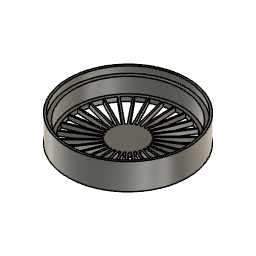
Fan front body (Autodesk Fusion 360 design; units mm, degrees)
Autodesk Fusion 360 part; units mm, degrees
sketch "Sketch1" plane through (0, 0, 0) normal (0, 0, 1) x (1, 0, 0) in component "P1"
  circle A0 centre (0, 0) radius 25
  circle A1 centre (0, 0) radius 137.5
  line L0 (-92.5259, 72.6579) -> (-105.6105, 51.8329)
  line L1 (-105.6105, 51.8329) -> (-114.0793, 28.7426)
  line L2 (-114.0793, 28.7426) -> (-117.5623, 4.3961)
  line L3 (-117.5623, 4.3961) -> (-115.9073, -20.1426)
  line L4 (-115.9073, -20.1426) -> (-109.1866, -43.8009)
  line L5 (-109.1866, -43.8009) -> (-97.6939, -65.5449)
  line L6 (-97.6939, -65.5449) -> (-81.9315, -84.4243)
  line L7 (-81.9315, -84.4243) -> (-62.5883, -99.6139)
  line L8 (-62.5883, -99.6139) -> (-40.5097, -110.4499)
  line L9 (-40.5097, -110.4499) -> (-16.6606, -116.4588)
  line L10 (-16.6606, -116.4588) -> (7.9166, -117.3778)
  line L11 (7.9166, -117.3778) -> (32.1478, -113.1669)
  line L12 (32.1478, -113.1669) -> (54.974, -104.01)
  line L13 (54.974, -104.01) -> (75.3976, -90.3074)
  line L14 (75.3976, -90.3074) -> (92.5259, -72.6579)
  line L15 (92.5259, -72.6579) -> (105.6105, -51.8329)
  line L16 (105.6105, -51.8329) -> (114.0793, -28.7426)
  line L17 (114.0793, -28.7426) -> (117.5623, -4.3961)
  line L18 (117.5623, -4.3961) -> (115.9073, 20.1426)
  line L19 (115.9073, 20.1426) -> (109.1866, 43.8009)
  line L20 (109.1866, 43.8009) -> (97.6939, 65.5449)
  line L21 (97.6939, 65.5449) -> (81.9315, 84.4243)
  line L22 (81.9315, 84.4243) -> (62.5883, 99.6139)
  line L23 (62.5883, 99.6139) -> (40.5097, 110.4499)
  line L24 (40.5097, 110.4499) -> (16.6606, 116.4588)
  line L25 (16.6606, 116.4588) -> (-7.9166, 117.3778)
  line L26 (-7.9166, 117.3778) -> (-32.1478, 113.1669)
  line L27 (-32.1478, 113.1669) -> (-54.974, 104.01)
  line L28 (-54.974, 104.01) -> (-75.3976, 90.3074)
  line L29 (-75.3976, 90.3074) -> (-92.5259, 72.6579)
  line L30 (-114.0793, 28.7426) -> (-117.5623, 4.3961)
  line L31 (-117.5623, 4.3961) -> (-115.9073, -20.1426)
  line L32 (-115.9073, -20.1426) -> (-109.1866, -43.8009)
  line L33 (-109.1866, -43.8009) -> (-97.6939, -65.5449)
  line L34 (-97.6939, -65.5449) -> (-81.9315, -84.4243)
  line L35 (-81.9315, -84.4243) -> (-62.5883, -99.6139)
  line L36 (-62.5883, -99.6139) -> (-40.5097, -110.4499)
  line L37 (-40.5097, -110.4499) -> (-16.6606, -116.4588)
  line L38 (-16.6606, -116.4588) -> (7.9166, -117.3778)
  line L39 (7.9166, -117.3778) -> (32.1478, -113.1669)
  line L40 (32.1478, -113.1669) -> (54.974, -104.01)
  line L41 (54.974, -104.01) -> (75.3976, -90.3074)
  line L42 (75.3976, -90.3074) -> (92.5259, -72.6579)
  line L43 (92.5259, -72.6579) -> (105.6105, -51.8329)
  line L44 (105.6105, -51.8329) -> (114.0793, -28.7426)
  line L45 (114.0793, -28.7426) -> (117.5623, -4.3961)
  line L46 (117.5623, -4.3961) -> (115.9073, 20.1426)
  line L47 (115.9073, 20.1426) -> (109.1866, 43.8009)
  line L48 (109.1866, 43.8009) -> (97.6939, 65.5449)
  line L49 (97.6939, 65.5449) -> (81.9315, 84.4243)
  line L50 (81.9315, 84.4243) -> (62.5883, 99.6139)
  line L51 (62.5883, 99.6139) -> (40.5097, 110.4499)
  line L52 (40.5097, 110.4499) -> (16.6606, 116.4588)
  line L53 (16.6606, 116.4588) -> (-7.9166, 117.3778)
  line L54 (-7.9166, 117.3778) -> (-32.1478, 113.1669)
  line L55 (-32.1478, 113.1669) -> (-54.974, 104.01)
  line L56 (-54.974, 104.01) -> (-75.3976, 90.3074)
  line L57 (-75.3976, 90.3074) -> (-92.5259, 72.6579)
  line L58 (-92.5259, 72.6579) -> (-105.6105, 51.8329)
  line L59 (-105.6105, 51.8329) -> (-114.0793, 28.7426)
  line L60 (-31.5682, 24.9223) -> (-36.06, 17.8143)
  line L61 (-36.06, 17.8143) -> (-38.9758, 9.9277)
  line L62 (-38.9758, 9.9277) -> (-40.1882, 1.6072)
  line L63 (-40.1882, 1.6072) -> (-39.6442, -6.7835)
  line L64 (-39.6442, -6.7835) -> (-37.3675, -14.8777)
  line L65 (-37.3675, -14.8777) -> (-33.4576, -22.3218)
  line L66 (-33.4576, -22.3218) -> (-28.0856, -28.7902)
  line L67 (-28.0856, -28.7902) -> (-21.486, -34.0004)
  line L68 (-21.486, -34.0004) -> (-13.9474, -37.7246)
  line L69 (-13.9474, -37.7246) -> (-5.7992, -39.8001)
  line L70 (-5.7992, -39.8001) -> (2.6024, -40.1361)
  line L71 (2.6024, -40.1361) -> (10.8903, -38.7179)
  line L72 (10.8903, -38.7179) -> (18.7022, -35.6076)
  line L73 (18.7022, -35.6076) -> (25.6968, -30.9411)
  line L74 (25.6968, -30.9411) -> (31.5682, -24.9223)
  line L75 (31.5682, -24.9223) -> (36.06, -17.8143)
  line L76 (36.06, -17.8143) -> (38.9758, -9.9277)
  line L77 (38.9758, -9.9277) -> (40.1882, -1.6072)
  line L78 (40.1882, -1.6072) -> (39.6442, 6.7835)
  line L79 (39.6442, 6.7835) -> (37.3675, 14.8777)
  line L80 (37.3675, 14.8777) -> (33.4576, 22.3218)
  line L81 (33.4576, 22.3218) -> (28.0856, 28.7902)
  line L82 (28.0856, 28.7902) -> (21.486, 34.0004)
  line L83 (21.486, 34.0004) -> (13.9474, 37.7246)
  line L84 (13.9474, 37.7246) -> (5.7992, 39.8001)
  line L85 (5.7992, 39.8001) -> (-2.6024, 40.1361)
  line L86 (-2.6024, 40.1361) -> (-10.8903, 38.7179)
  line L87 (-10.8903, 38.7179) -> (-18.7022, 35.6076)
  line L88 (-18.7022, 35.6076) -> (-25.6968, 30.9411)
  line L89 (-25.6968, 30.9411) -> (-31.5682, 24.9223)
  line L90 (-105.6105, 51.8329) -> (-36.06, 17.8143)
  line L91 (-114.0793, 28.7426) -> (-38.9758, 9.9277)
  line L92 (-117.5623, 4.3961) -> (-40.1882, 1.6072)
  line L93 (-115.9073, -20.1426) -> (-39.6442, -6.7835)
  line L94 (-109.1866, -43.8009) -> (-37.3675, -14.8777)
  line L95 (-97.6939, -65.5449) -> (-33.4576, -22.3218)
  line L96 (-28.0856, -28.7902) -> (-81.9315, -84.4243)
  line L97 (-62.5883, -99.6139) -> (-21.486, -34.0004)
  line L98 (-13.9474, -37.7246) -> (-40.5097, -110.4499)
  line L99 (-5.7992, -39.8001) -> (-16.6606, -116.4588)
  line L100 (2.6024, -40.1361) -> (7.9166, -117.3778)
  line L101 (10.8903, -38.7179) -> (32.1478, -113.1669)
  line L102 (18.7022, -35.6076) -> (54.974, -104.01)
  line L103 (25.6968, -30.9411) -> (75.3976, -90.3074)
  line L104 (31.5682, -24.9223) -> (92.5259, -72.6579)
  line L105 (36.06, -17.8143) -> (105.6105, -51.8329)
  line L106 (38.9758, -9.9277) -> (114.0793, -28.7426)
  line L107 (40.1882, -1.6072) -> (117.5623, -4.3961)
  line L108 (39.6442, 6.7835) -> (115.9073, 20.1426)
  line L109 (37.3675, 14.8777) -> (109.1866, 43.8009)
  line L110 (33.4576, 22.3218) -> (97.6939, 65.5449)
  line L111 (28.0856, 28.7902) -> (81.9315, 84.4243)
  line L112 (21.486, 34.0004) -> (62.5883, 99.6139)
  line L113 (13.9474, 37.7246) -> (40.5097, 110.4499)
  line L114 (16.6606, 116.4588) -> (5.7992, 39.8001)
  line L115 (-7.9166, 117.3778) -> (-2.6024, 40.1361)
  line L116 (-32.1478, 113.1669) -> (-10.8903, 38.7179)
  line L117 (-54.974, 104.01) -> (-18.7022, 35.6076)
  line L118 (-92.5259, 72.6579) -> (-31.5682, 24.9223)
  line L119 (-75.3976, 90.3074) -> (-25.6968, 30.9411)
  dimension "d1" = 50
  dimension "d6" = 275
  dimension "d7" = 117
  dimension "d8" = 40
  constraint coincident A0.centre A1.centre
  measures "d1" diameter of A0
  measures "d6" diameter of A1
  measures "d7" distance of A0.centre L29
  measures "d8" distance of A0.centre L89
sketch "Sketch2" plane through (0, 0, 0) normal (0, 0, 1) x (1, 0, 0) in component "P1"
  line L0 (-36.3108, 17.2975) -> (-39.1136, 9.3701)
  line L1 (-39.1136, 9.3701) -> (-40.2071, 1.0331)
  line L2 (-40.2071, 1.0331) -> (-39.5432, -7.349)
  line L3 (-39.5432, -7.349) -> (-37.1512, -15.4099)
  line L4 (-37.1512, -15.4099) -> (-33.1355, -22.7973)
  line L5 (-33.1355, -22.7973) -> (-27.6715, -29.1884)
  line L6 (-27.6715, -29.1884) -> (-20.9983, -34.3038)
  line L7 (-20.9983, -34.3038) -> (-13.4072, -37.9199)
  line L8 (-13.4072, -37.9199) -> (-5.2303, -39.8788)
  line L9 (-5.2303, -39.8788) -> (3.1753, -40.0948)
  line L10 (3.1753, -40.0948) -> (11.4421, -38.5584)
  line L11 (11.4421, -38.5584) -> (19.2088, -35.3369)
  line L12 (19.2088, -35.3369) -> (26.136, -30.571)
  line L13 (26.136, -30.571) -> (31.9209, -24.4689)
  line L14 (31.9209, -24.4689) -> (36.3108, -17.2975)
  line L15 (36.3108, -17.2975) -> (39.1136, -9.3701)
  line L16 (39.1136, -9.3701) -> (40.2071, -1.0331)
  line L17 (40.2071, -1.0331) -> (39.5432, 7.349)
  line L18 (39.5432, 7.349) -> (37.1512, 15.4099)
  line L19 (37.1512, 15.4099) -> (33.1355, 22.7973)
  line L20 (33.1355, 22.7973) -> (27.6715, 29.1884)
  line L21 (27.6715, 29.1884) -> (20.9983, 34.3038)
  line L22 (20.9983, 34.3038) -> (13.4072, 37.9199)
  line L23 (13.4072, 37.9199) -> (5.2303, 39.8788)
  line L24 (5.2303, 39.8788) -> (-3.1753, 40.0948)
  line L25 (-3.1753, 40.0948) -> (-11.4421, 38.5584)
  line L26 (-11.4421, 38.5584) -> (-19.2088, 35.3369)
  line L27 (-19.2088, 35.3369) -> (-26.136, 30.571)
  line L28 (-26.136, 30.571) -> (-31.9209, 24.4689)
  line L29 (-31.9209, 24.4689) -> (-36.3108, 17.2975)
  line L30 (-94.5441, 70.4382) -> (-34.1158, 20.8832)
  line L31 (-31.9209, 24.4689) -> (-91.7989, 73.5727)
  line L32 (-91.7989, 73.5727) -> (-94.5441, 70.4382)
  line L33 (-75.334, 90.2327) -> (-77.6493, 88.325)
  line L34 (-77.6493, 88.325) -> (-29.0285, 27.52)
  line L35 (-26.136, 30.571) -> (-75.334, 90.2327)
  line L36 (-94.5441, 70.4382) -> (-93.1715, 72.0054)
  line L37 (-57.7827, 102.4024) -> (-55.0494, 103.6389)
  line L38 (-55.0494, 103.6389) -> (-19.2088, 35.3369)
  line L39 (-22.6724, 32.9539) -> (-57.7827, 102.4024)
  line L40 (-32.148, 113.167) -> (-34.9624, 112.1282)
  line L41 (-34.9624, 112.1282) -> (-15.3254, 36.9477)
  line L42 (-11.4421, 38.5584) -> (-32.148, 113.167)
  line L43 (-3.1753, 40.0948) -> (-7.7901, 117.2299)
  line L44 (-7.7901, 117.2299) -> (-10.7847, 117.0508)
  line L45 (-10.7847, 117.0508) -> (-7.3087, 39.3266)
  line L46 (-3.1753, 40.0948) -> (-7.7901, 117.2299)
  line L47 (16.8251, 116.2807) -> (13.8251, 116.2807)
  line L48 (13.8251, 116.2807) -> (1.0275, 39.9868)
  line L49 (5.2303, 39.8788) -> (16.8251, 116.2807)
  line L50 (40.5383, 110.4147) -> (37.6703, 111.2947)
  line L51 (37.6703, 111.2947) -> (9.3188, 38.8994)
  line L52 (13.4072, 37.9199) -> (40.5383, 110.4147)
  line L53 (62.5134, 99.4538) -> (59.7037, 100.5053)
  line L54 (59.7037, 100.5053) -> (17.2027, 36.1118)
  line L55 (20.9983, 34.3038) -> (62.5134, 99.4538)
  line L56 (82, 84) -> (79.7982, 86.0377)
  line L57 (79.7982, 86.0377) -> (24.3349, 31.7461)
  line L58 (27.6715, 29.1884) -> (82, 84)
  line L59 (97.7404, 65.3757) -> (95.6097, 67.4876)
  line L60 (95.6097, 67.4876) -> (30.4035, 25.9928)
  line L61 (33.1355, 22.7973) -> (97.7404, 65.3757)
  line L62 (109.2924, 44.0865) -> (107.6415, 46.5914)
  line L63 (107.6415, 46.5914) -> (35.1433, 19.1036)
  line L64 (37.1512, 15.4099) -> (109.2924, 44.0865)
  line L65 (116, 20) -> (114.8918, 22.7878)
  line L66 (114.8918, 22.7878) -> (38.3472, 11.3794)
  line L67 (39.5432, 7.349) -> (116, 20)
  line L68 (117.789, -4.8117) -> (117.2992, -1.8519)
  line L69 (117.2992, -1.8519) -> (39.8752, 3.1579)
  line L70 (40.2071, -1.0331) -> (117.789, -4.8117)
  line L71 (114, -29) -> (114.4863, -26.0397)
  line L72 (114.4863, -26.0397) -> (39.6603, -5.2016)
  line L73 (39.1136, -9.3701) -> (114, -29)
  line L74 (105.7119, -51.9678) -> (106.4726, -49.0659)
  line L75 (106.4726, -49.0659) -> (37.7122, -13.3338)
  line L76 (36.3108, -17.2975) -> (105.7119, -51.9678)
  line L77 (92.7602, -72.7218) -> (94.1009, -70.038)
  line L78 (94.1009, -70.038) -> (34.1158, -20.8832)
  line L79 (31.9209, -24.4689) -> (92.7602, -72.7218)
  line L80 (75.4679, -90.2781) -> (77.7305, -88.3082)
  line L81 (77.7305, -88.3082) -> (29.0285, -27.52)
  line L82 (26.136, -30.571) -> (75.4679, -90.2781)
  line L83 (32.3249, -113.2073) -> (35.0941, -112.0535)
  line L84 (35.0941, -112.0535) -> (15.3254, -36.9477)
  line L85 (11.4421, -38.5584) -> (32.3249, -113.2073)
  line L86 (55, -104) -> (57.5118, -102.3596)
  line L87 (57.5118, -102.3596) -> (22.6724, -32.9539)
  line L88 (19.2088, -35.3369) -> (55, -104)
  line L89 (7.3087, -117.1355) -> (10.2582, -116.5873)
  line L90 (10.2582, -116.5873) -> (7.3087, -39.3266)
  line L91 (3.1753, -40.0948) -> (7.3087, -117.1355)
  line L92 (-16.4966, -116.6928) -> (-13.4966, -116.6928)
  line L93 (-13.4966, -116.6928) -> (-1.0275, -39.9868)
  line L94 (-5.2303, -39.8788) -> (-16.4966, -116.6928)
  line L95 (-40, -110) -> (-37.1974, -111.0702)
  line L96 (-37.1974, -111.0702) -> (-9.3188, -38.8994)
  line L97 (-13.4072, -37.9199) -> (-40, -110)
  line L98 (-62.5344, -99.65) -> (-59.7198, -100.6884)
  line L99 (-59.7198, -100.6884) -> (-17.2027, -36.1118)
  line L100 (-20.9983, -34.3038) -> (-62.5344, -99.65)
  line L101 (-82.0119, -84.3778) -> (-79.5062, -86.0276)
  line L102 (-79.5062, -86.0276) -> (-24.3349, -31.7461)
  line L103 (-27.6715, -29.1884) -> (-82.0119, -84.3778)
  line L104 (-97.7267, -65.5643) -> (-95.589, -67.6691)
  line L105 (-95.589, -67.6691) -> (-30.4035, -25.9928)
  line L106 (-33.1355, -22.7973) -> (-97.7267, -65.5643)
  line L107 (-109.2361, -44.1808) -> (-107.5799, -46.6822)
  line L108 (-107.5799, -46.6822) -> (-35.1433, -19.1036)
  line L109 (-37.1512, -15.4099) -> (-109.2361, -44.1808)
  line L110 (-116, -20) -> (-114.8879, -22.7863)
  line L111 (-114.8879, -22.7863) -> (-38.3472, -11.3794)
  line L112 (-39.5432, -7.349) -> (-116, -20)
  line L113 (-117.8376, 4.2071) -> (-117.3479, 1.2473)
  line L114 (-117.3479, 1.2473) -> (-39.8752, -3.1579)
  line L115 (-40.2071, 1.0331) -> (-117.8376, 4.2071)
  line L116 (-114.3122, 28.3563) -> (-114.4825, 25.3611)
  line L117 (-114.4825, 25.3611) -> (-39.6603, 5.2016)
  line L118 (-39.1136, 9.3701) -> (-114.3122, 28.3563)
  line L119 (-105.3224, 51.9766) -> (-106.1029, 49.0799)
  line L120 (-106.1029, 49.0799) -> (-37.7122, 13.3338)
  line L121 (-36.3108, 17.2975) -> (-105.3224, 51.9766)
  point P0 (-75.3976, 90.3074)
  point P1 (-92.5259, 72.6579)
  dimension "d9" = 40
  dimension "d10" = 3
  dimension "d11" = 3
  dimension "d12" = 3
  dimension "d13" = 3
  dimension "d14" = 3
  dimension "d16" = 3
  dimension "d17" = 3
  dimension "d18" = 3
  dimension "d19" = 3
  dimension "d20" = 3
  dimension "d21" = 3
  dimension "d22" = 3
  dimension "d23" = 3
  dimension "d24" = 3
  dimension "d25" = 3
  dimension "d26" = 3
  dimension "d27" = 3
  dimension "d28" = 3
  dimension "d29" = 3
  dimension "d30" = 3
  dimension "d31" = 3
  dimension "d32" = 3
  dimension "d33" = 3
  dimension "d34" = 3
  dimension "d35" = 3
  dimension "d36" = 3
  dimension "d37" = 3
  dimension "d38" = 3
  dimension "d39" = 3
  dimension "d40" = 3
  dimension "d41" = 3
  constraint midpoint L29 L30.end
  constraint parallel L30 L31
  constraint midpoint L28 L34.end
  constraint midpoint L32 L36.end
  constraint midpoint L27 L39.start
  constraint midpoint L26 L41.end
  constraint perpendicular L43 L44
  constraint midpoint L25 L45.end
  constraint horizontal L47
  constraint midpoint L24 L48.end
  constraint midpoint L23 L51.end
  constraint perpendicular L52 L53
  constraint midpoint L22 L54.end
  constraint midpoint L21 L57.end
  constraint perpendicular L58 L59
  constraint midpoint L20 L60.end
  constraint perpendicular L61 L62
  constraint midpoint L19 L63.end
  constraint perpendicular L64 L65
  constraint midpoint L18 L66.end
  constraint perpendicular L67 L68
  constraint midpoint L17 L69.end
  constraint midpoint L16 L72.end
  constraint perpendicular L73 L74
  constraint midpoint L15 L75.end
  constraint perpendicular L76 L77
  constraint midpoint L14 L78.end
  constraint midpoint L13 L81.end
  constraint midpoint L11 L84.end
  constraint midpoint L12 L87.end
  constraint parallel L10 L89
  constraint midpoint L10 L90.end
  constraint horizontal L92
  constraint midpoint L9 L93.end
  constraint midpoint L8 L96.end
  constraint perpendicular L97 L98
  constraint midpoint L7 L99.end
  constraint perpendicular L99 L101
  constraint midpoint L6 L102.end
  constraint perpendicular L103 L104
  constraint midpoint L5 L105.end
  constraint perpendicular L106 L107
  constraint midpoint L4 L108.end
  constraint perpendicular L109 L110
  constraint midpoint L3 L111.end
  constraint perpendicular L112 L113
  constraint midpoint L2 L114.end
  constraint perpendicular L114 L116
  constraint midpoint L1 L117.end
  constraint perpendicular L117 L119
  constraint midpoint L0 L120.end
  measures "d9" distance of origin L29
  measures "d10" distance of L33.start L33.end
  measures "d11" distance of L33.end P0
  measures "d12" distance of L30.start P1
  measures "d13" distance of L37.start L37.end
  measures "d14" distance of L40.start L40.end
  measures "d16" distance of L43.end L44.end
  measures "d17" distance of L47.start L47.end
  measures "d18" distance of L50.start L50.end
  measures "d19" distance of L53.start L53.end
  measures "d20" distance of L56.start L56.end
  measures "d21" distance of L59.start L59.end
  measures "d22" distance of L62.start L62.end
  measures "d23" distance of L65.start L65.end
  measures "d24" distance of L68.start L68.end
  measures "d25" distance of L71.start L71.end
  measures "d26" distance of L74.start L74.end
  measures "d27" distance of L77.start L77.end
  measures "d28" distance of L80.start L80.end
  measures "d29" distance of L83.start L83.end
  measures "d30" distance of L86.start L86.end
  measures "d31" distance of L89.start L89.end
  measures "d32" distance of L92.start L92.end
  measures "d33" distance of L95.start L95.end
  measures "d34" distance of L98.start L98.end
  measures "d35" distance of L101.start L101.end
  measures "d36" distance of L104.start L104.end
  measures "d37" distance of L107.start L107.end
  measures "d38" distance of L110.start L110.end
  measures "d39" distance of L113.start L113.end
  measures "d40" distance of L116.start L116.end
  measures "d41" distance of L119.start L119.end
extrude "Extrude1" add sketch "Sketch2" sketch "Sketch1" along normal blind 10 of sketch 2 contours A1 in component "P1"
sketch "Sketch3" plane through (0, 0, 10) normal (0, 0, 1) x (-1, 0, 0) in component "P1"
  line L0 (114.4294, -26.2951) -> (114.4825, -25.3611)
  line L1 (114.4825, -25.3611) -> (39.6603, -5.2016)
  line L2 (39.6603, -5.2016) -> (40.2071, -1.0331)
  line L3 (40.2071, -1.0331) -> (117.5488, -4.1953)
  line L4 (117.5488, -4.1953) -> (117.5623, -4.3961)
  line L5 (117.5623, -4.3961) -> (114.4294, -26.2951)
  line L6 (117.3513, -1.268) -> (117.3479, -1.2473)
  line L7 (117.3479, -1.2473) -> (39.8752, 3.1579)
  line L8 (39.8752, 3.1579) -> (39.5432, 7.349)
  line L9 (39.5432, 7.349) -> (115.9178, 19.9864)
  line L10 (115.9178, 19.9864) -> (117.3513, -1.268)
  line L11 (115.8188, 20.4539) -> (114.8879, 22.7863)
  line L12 (114.8879, 22.7863) -> (38.3472, 11.3794)
  line L13 (38.3472, 11.3794) -> (37.1512, 15.4099)
  line L14 (37.1512, 15.4099) -> (109.0294, 44.0983)
  line L15 (109.0294, 44.0983) -> (109.1866, 43.8009)
  line L16 (109.1866, 43.8009) -> (115.8188, 20.4539)
  line L17 (107.9951, 46.0551) -> (107.5799, 46.6822)
  line L18 (107.5799, 46.6822) -> (35.1433, 19.1036)
  line L19 (35.1433, 19.1036) -> (33.1355, 22.7973)
  line L20 (33.1355, 22.7973) -> (97.6947, 65.5432)
  line L21 (97.6947, 65.5432) -> (107.9951, 46.0551)
  line L22 (97.451, 65.8357) -> (95.589, 67.6691)
  line L23 (95.589, 67.6691) -> (30.4035, 25.9928)
  line L24 (30.4035, 25.9928) -> (27.6715, 29.1884)
  line L25 (27.6715, 29.1884) -> (81.9893, 84.355)
  line L26 (81.9893, 84.355) -> (97.451, 65.8357)
  line L27 (81.8802, 84.4645) -> (79.5062, 86.0276)
  line L28 (79.5062, 86.0276) -> (24.3349, 31.7461)
  line L29 (24.3349, 31.7461) -> (20.9983, 34.3038)
  line L30 (20.9983, 34.3038) -> (62.5297, 99.6426)
  line L31 (62.5297, 99.6426) -> (62.5883, 99.6139)
  line L32 (62.5883, 99.6139) -> (81.8802, 84.4645)
  line L33 (62.4555, 99.6791) -> (59.7198, 100.6884)
  line L34 (59.7198, 100.6884) -> (17.2027, 36.1118)
  line L35 (17.2027, 36.1118) -> (13.4072, 37.9199)
  line L36 (13.4072, 37.9199) -> (40, 110)
  line L37 (40, 110) -> (37.1974, 111.0702)
  line L38 (37.1974, 111.0702) -> (9.3188, 38.8994)
  line L39 (9.3188, 38.8994) -> (5.2303, 39.8788)
  line L40 (5.2303, 39.8788) -> (16.4634, 116.4661)
  line L41 (16.4634, 116.4661) -> (16.6606, 116.4588)
  line L42 (16.6606, 116.4588) -> (40.5097, 110.4499)
  line L43 (40.5097, 110.4499) -> (62.4555, 99.6791)
  line L44 (13.4779, 116.5778) -> (1.0275, 39.9868)
  line L45 (1.0275, 39.9868) -> (-3.1753, 40.0948)
  line L46 (-3.1753, 40.0948) -> (-7.3087, 117.1355)
  line L47 (-7.3087, 117.1355) -> (-10.2582, 116.5873)
  line L48 (-10.2582, 116.5873) -> (-7.3087, 39.3266)
  line L49 (-7.3087, 39.3266) -> (-11.4421, 38.5584)
  line L50 (-11.4421, 38.5584) -> (-32.2969, 113.1071)
  line L51 (-32.2969, 113.1071) -> (-32.1478, 113.1669)
  line L52 (-32.1478, 113.1669) -> (-7.9166, 117.3778)
  line L53 (-7.9166, 117.3778) -> (13.4779, 116.5778)
  line L54 (-35.0778, 111.9915) -> (-15.3254, 36.9477)
  line L55 (-15.3254, 36.9477) -> (-19.2088, 35.3369)
  line L56 (-19.2088, 35.3369) -> (-54.9971, 103.9945)
  line L57 (-54.9971, 103.9945) -> (-54.974, 104.01)
  line L58 (-54.974, 104.01) -> (-35.0778, 111.9915)
  line L59 (-57.4922, 102.3205) -> (-22.6724, 32.9539)
  line L60 (-22.6724, 32.9539) -> (-26.136, 30.571)
  line L61 (-26.136, 30.571) -> (-75.4486, 90.2548)
  line L62 (-75.4486, 90.2548) -> (-75.3976, 90.3074)
  line L63 (-75.3976, 90.3074) -> (-57.4922, 102.3205)
  line L64 (-77.5529, 88.0865) -> (-29.0285, 27.52)
  line L65 (-29.0285, 27.52) -> (-31.9209, 24.4689)
  line L66 (-31.9209, 24.4689) -> (-92.5771, 72.5765)
  line L67 (-92.5771, 72.5765) -> (-92.5259, 72.6579)
  line L68 (-92.5259, 72.6579) -> (-77.5529, 88.0865)
  line L69 (-93.8248, 70.5906) -> (-94.1009, 70.038)
  line L70 (-94.1009, 70.038) -> (-34.1158, 20.8832)
  line L71 (-34.1158, 20.8832) -> (-36.3108, 17.2975)
  line L72 (-36.3108, 17.2975) -> (-105.5702, 51.897)
  line L73 (-105.5702, 51.897) -> (-93.8248, 70.5906)
  line L74 (-114.0123, 28.9253) -> (-114.3288, 26.9982)
  line L75 (-114.3288, 26.9982) -> (-114.0793, 28.7426)
  line L76 (-114.0793, 28.7426) -> (-114.0123, 28.9253)
  line L77 (-113.9862, 28.9964) -> (-106.09, 50.5256)
  line L78 (-106.09, 50.5256) -> (-106.4726, 49.0659)
  line L79 (-106.4726, 49.0659) -> (-37.7122, 13.3338)
  line L80 (-37.7122, 13.3338) -> (-39.1136, 9.3701)
  line L81 (-39.1136, 9.3701) -> (-113.9862, 28.9964)
  line L82 (-114.4667, 26.0342) -> (-39.6603, 5.2016)
  line L83 (-39.6603, 5.2016) -> (-40.2071, 1.0331)
  line L84 (-40.2071, 1.0331) -> (-117.5048, 4.7978)
  line L85 (-117.5048, 4.7978) -> (-114.4667, 26.0342)
  line L86 (-117.4537, 2.7851) -> (-117.2992, 1.8519)
  line L87 (-117.2992, 1.8519) -> (-39.8752, -3.1579)
  line L88 (-39.8752, -3.1579) -> (-39.5432, -7.349)
  line L89 (-39.5432, -7.349) -> (-115.9178, -19.9864)
  line L90 (-115.9178, -19.9864) -> (-117.4537, 2.7851)
  line L91 (-115.817, -20.4604) -> (-114.8918, -22.7878)
  line L92 (-114.8918, -22.7878) -> (-38.3472, -11.3794)
  line L93 (-38.3472, -11.3794) -> (-37.1512, -15.4099)
  line L94 (-37.1512, -15.4099) -> (-109.0802, -44.0021)
  line L95 (-109.0802, -44.0021) -> (-109.1866, -43.8009)
  line L96 (-109.1866, -43.8009) -> (-115.817, -20.4604)
  line L97 (-107.9955, -46.0543) -> (-107.6415, -46.5914)
  line L98 (-107.6415, -46.5914) -> (-35.1433, -19.1036)
  line L99 (-35.1433, -19.1036) -> (-33.1355, -22.7973)
  line L100 (-33.1355, -22.7973) -> (-97.7404, -65.3757)
  line L101 (-97.7404, -65.3757) -> (-95.6097, -67.4876)
  line L102 (-95.6097, -67.4876) -> (-30.4035, -25.9928)
  line L103 (-30.4035, -25.9928) -> (-27.6715, -29.1884)
  line L104 (-27.6715, -29.1884) -> (-82, -84)
  line L105 (-82, -84) -> (-79.7982, -86.0377)
  line L106 (-79.7982, -86.0377) -> (-24.3349, -31.7461)
  line L107 (-24.3349, -31.7461) -> (-20.9983, -34.3038)
  line L108 (-20.9983, -34.3038) -> (-62.5134, -99.4538)
  line L109 (-62.5134, -99.4538) -> (-59.7037, -100.5053)
  line L110 (-59.7037, -100.5053) -> (-17.2027, -36.1118)
  line L111 (-17.2027, -36.1118) -> (-13.4072, -37.9199)
  line L112 (-13.4072, -37.9199) -> (-40.5383, -110.4147)
  line L113 (-40.5383, -110.4147) -> (-40.0275, -110.5714)
  line L114 (-40.0275, -110.5714) -> (-40.5097, -110.4499)
  line L115 (-40.5097, -110.4499) -> (-62.5883, -99.6139)
  line L116 (-62.5883, -99.6139) -> (-81.9315, -84.4243)
  line L117 (-81.9315, -84.4243) -> (-97.6939, -65.5449)
  line L118 (-97.6939, -65.5449) -> (-107.9955, -46.0543)
  line L119 (-37.6242, -111.1769) -> (-9.3188, -38.8994)
  line L120 (-9.3188, -38.8994) -> (-5.2303, -39.8788)
  line L121 (-5.2303, -39.8788) -> (-16.8251, -116.2807)
  line L122 (-16.8251, -116.2807) -> (-13.8251, -116.2807)
  line L123 (-13.8251, -116.2807) -> (-1.0275, -39.9868)
  line L124 (-1.0275, -39.9868) -> (3.1753, -40.0948)
  line L125 (3.1753, -40.0948) -> (7.7901, -117.2299)
  line L126 (7.7901, -117.2299) -> (9.2805, -117.1408)
  line L127 (9.2805, -117.1408) -> (7.9166, -117.3778)
  line L128 (7.9166, -117.3778) -> (-16.6606, -116.4588)
  line L129 (-16.6606, -116.4588) -> (-37.6242, -111.1769)
  line L130 (10.7771, -116.8807) -> (7.3087, -39.3266)
  line L131 (7.3087, -39.3266) -> (11.4421, -38.5584)
  line L132 (11.4421, -38.5584) -> (32.1479, -113.1668)
  line L133 (32.1479, -113.1668) -> (32.1478, -113.1669)
  line L134 (32.1478, -113.1669) -> (10.7771, -116.8807)
  line L135 (34.941, -112.0464) -> (15.3254, -36.9477)
  line L136 (15.3254, -36.9477) -> (19.2088, -35.3369)
  line L137 (19.2088, -35.3369) -> (55.0494, -103.6389)
  line L138 (55.0494, -103.6389) -> (56.5162, -102.9753)
  line L139 (56.5162, -102.9753) -> (54.974, -104.01)
  line L140 (54.974, -104.01) -> (34.941, -112.0464)
  line L141 (57.6782, -102.1957) -> (22.6724, -32.9539)
  line L142 (22.6724, -32.9539) -> (26.136, -30.571)
  line L143 (26.136, -30.571) -> (75.334, -90.2327)
  line L144 (75.334, -90.2327) -> (76.0131, -89.6732)
  line L145 (76.0131, -89.6732) -> (75.3976, -90.3074)
  line L146 (75.3976, -90.3074) -> (57.6782, -102.1957)
  line L147 (77.5012, -88.1398) -> (29.0285, -27.52)
  line L148 (29.0285, -27.52) -> (31.9209, -24.4689)
  line L149 (31.9209, -24.4689) -> (91.7094, -73.4993)
  line L150 (91.7094, -73.4993) -> (77.5012, -88.1398)
  line L151 (114.1408, -28.313) -> (114.0793, -28.7426)
  line L152 (114.0793, -28.7426) -> (105.6105, -51.8329)
  line L153 (105.6105, -51.8329) -> (94.1326, -70.1008)
  line L154 (94.1326, -70.1008) -> (34.1158, -20.8832)
  line L155 (34.1158, -20.8832) -> (36.3108, -17.2975)
  line L156 (36.3108, -17.2975) -> (105.3224, -51.9766)
  line L157 (105.3224, -51.9766) -> (106.1029, -49.0799)
  line L158 (106.1029, -49.0799) -> (37.7122, -13.3338)
  line L159 (37.7122, -13.3338) -> (39.1136, -9.3701)
  line L160 (39.1136, -9.3701) -> (114.1408, -28.313)
  circle A0 centre (0, 0) radius 137.5
  circle A1 centre (0, 0) radius 137.5
  circle A2 centre (0, 0) radius 126.4911
  dimension "d44" = 275
  constraint concentric A0 A1
  constraint coincident A0.centre A1.centre
  measures "d44" diameter of A1
extrude "Extrude2" add sketch "Sketch3" along normal blind 50 contours A0 A1 in component "P1"
sketch "Sketch4" plane through (0, 0, 10) normal (0, 0, 1) x (-1, 0, 0) in component "P1"
  circle A0 centre (0, 0) radius 126.4911
  line L0 (114.4294, -26.2951) -> (114.4825, -25.3611)
  line L1 (114.4825, -25.3611) -> (39.6603, -5.2016)
  line L2 (39.6603, -5.2016) -> (40.2071, -1.0331)
  line L3 (40.2071, -1.0331) -> (117.5488, -4.1953)
  line L4 (117.5488, -4.1953) -> (117.5623, -4.3961)
  line L5 (117.5623, -4.3961) -> (114.4294, -26.2951)
  line L6 (117.3513, -1.268) -> (117.3479, -1.2473)
  line L7 (117.3479, -1.2473) -> (39.8752, 3.1579)
  line L8 (39.8752, 3.1579) -> (39.5432, 7.349)
  line L9 (39.5432, 7.349) -> (115.9178, 19.9864)
  line L10 (115.9178, 19.9864) -> (117.3513, -1.268)
  line L11 (115.8188, 20.4539) -> (114.8879, 22.7863)
  line L12 (114.8879, 22.7863) -> (38.3472, 11.3794)
  line L13 (38.3472, 11.3794) -> (37.1512, 15.4099)
  line L14 (37.1512, 15.4099) -> (109.0294, 44.0983)
  line L15 (109.0294, 44.0983) -> (109.1866, 43.8009)
  line L16 (109.1866, 43.8009) -> (115.8188, 20.4539)
  line L17 (107.9951, 46.0551) -> (107.5799, 46.6822)
  line L18 (107.5799, 46.6822) -> (35.1433, 19.1036)
  line L19 (35.1433, 19.1036) -> (33.1355, 22.7973)
  line L20 (33.1355, 22.7973) -> (97.6947, 65.5432)
  line L21 (97.6947, 65.5432) -> (107.9951, 46.0551)
  line L22 (97.451, 65.8357) -> (95.589, 67.6691)
  line L23 (95.589, 67.6691) -> (30.4035, 25.9928)
  line L24 (30.4035, 25.9928) -> (27.6715, 29.1884)
  line L25 (27.6715, 29.1884) -> (81.9893, 84.355)
  line L26 (81.9893, 84.355) -> (97.451, 65.8357)
  line L27 (81.8802, 84.4645) -> (79.5062, 86.0276)
  line L28 (79.5062, 86.0276) -> (24.3349, 31.7461)
  line L29 (24.3349, 31.7461) -> (20.9983, 34.3038)
  line L30 (20.9983, 34.3038) -> (62.5297, 99.6426)
  line L31 (62.5297, 99.6426) -> (62.5883, 99.6139)
  line L32 (62.5883, 99.6139) -> (81.8802, 84.4645)
  line L33 (62.4555, 99.6791) -> (59.7198, 100.6884)
  line L34 (59.7198, 100.6884) -> (17.2027, 36.1118)
  line L35 (17.2027, 36.1118) -> (13.4072, 37.9199)
  line L36 (13.4072, 37.9199) -> (40, 110)
  line L37 (40, 110) -> (37.1974, 111.0702)
  line L38 (37.1974, 111.0702) -> (9.3188, 38.8994)
  line L39 (9.3188, 38.8994) -> (5.2303, 39.8788)
  line L40 (5.2303, 39.8788) -> (16.4634, 116.4661)
  line L41 (16.4634, 116.4661) -> (16.6606, 116.4588)
  line L42 (16.6606, 116.4588) -> (40.5097, 110.4499)
  line L43 (40.5097, 110.4499) -> (62.4555, 99.6791)
  line L44 (13.4779, 116.5778) -> (1.0275, 39.9868)
  line L45 (1.0275, 39.9868) -> (-3.1753, 40.0948)
  line L46 (-3.1753, 40.0948) -> (-7.3087, 117.1355)
  line L47 (-7.3087, 117.1355) -> (-10.2582, 116.5873)
  line L48 (-10.2582, 116.5873) -> (-7.3087, 39.3266)
  line L49 (-7.3087, 39.3266) -> (-11.4421, 38.5584)
  line L50 (-11.4421, 38.5584) -> (-32.2969, 113.1071)
  line L51 (-32.2969, 113.1071) -> (-32.1478, 113.1669)
  line L52 (-32.1478, 113.1669) -> (-7.9166, 117.3778)
  line L53 (-7.9166, 117.3778) -> (13.4779, 116.5778)
  line L54 (-35.0778, 111.9915) -> (-15.3254, 36.9477)
  line L55 (-15.3254, 36.9477) -> (-19.2088, 35.3369)
  line L56 (-19.2088, 35.3369) -> (-54.9971, 103.9945)
  line L57 (-54.9971, 103.9945) -> (-54.974, 104.01)
  line L58 (-54.974, 104.01) -> (-35.0778, 111.9915)
  line L59 (-57.4922, 102.3205) -> (-22.6724, 32.9539)
  line L60 (-22.6724, 32.9539) -> (-26.136, 30.571)
  line L61 (-26.136, 30.571) -> (-75.4486, 90.2548)
  line L62 (-75.4486, 90.2548) -> (-75.3976, 90.3074)
  line L63 (-75.3976, 90.3074) -> (-57.4922, 102.3205)
  line L64 (-77.5529, 88.0865) -> (-29.0285, 27.52)
  line L65 (-29.0285, 27.52) -> (-31.9209, 24.4689)
  line L66 (-31.9209, 24.4689) -> (-92.5771, 72.5765)
  line L67 (-92.5771, 72.5765) -> (-92.5259, 72.6579)
  line L68 (-92.5259, 72.6579) -> (-77.5529, 88.0865)
  line L69 (-93.8248, 70.5906) -> (-94.1009, 70.038)
  line L70 (-94.1009, 70.038) -> (-34.1158, 20.8832)
  line L71 (-34.1158, 20.8832) -> (-36.3108, 17.2975)
  line L72 (-36.3108, 17.2975) -> (-105.5702, 51.897)
  line L73 (-105.5702, 51.897) -> (-93.8248, 70.5906)
  line L74 (-114.0123, 28.9253) -> (-114.3288, 26.9982)
  line L75 (-114.3288, 26.9982) -> (-114.0793, 28.7426)
  line L76 (-114.0793, 28.7426) -> (-114.0123, 28.9253)
  line L77 (-113.9862, 28.9964) -> (-106.09, 50.5256)
  line L78 (-106.09, 50.5256) -> (-106.4726, 49.0659)
  line L79 (-106.4726, 49.0659) -> (-37.7122, 13.3338)
  line L80 (-37.7122, 13.3338) -> (-39.1136, 9.3701)
  line L81 (-39.1136, 9.3701) -> (-113.9862, 28.9964)
  line L82 (-114.4667, 26.0342) -> (-39.6603, 5.2016)
  line L83 (-39.6603, 5.2016) -> (-40.2071, 1.0331)
  line L84 (-40.2071, 1.0331) -> (-117.5048, 4.7978)
  line L85 (-117.5048, 4.7978) -> (-114.4667, 26.0342)
  line L86 (-117.4537, 2.7851) -> (-117.2992, 1.8519)
  line L87 (-117.2992, 1.8519) -> (-39.8752, -3.1579)
  line L88 (-39.8752, -3.1579) -> (-39.5432, -7.349)
  line L89 (-39.5432, -7.349) -> (-115.9178, -19.9864)
  line L90 (-115.9178, -19.9864) -> (-117.4537, 2.7851)
  line L91 (-115.817, -20.4604) -> (-114.8918, -22.7878)
  line L92 (-114.8918, -22.7878) -> (-38.3472, -11.3794)
  line L93 (-38.3472, -11.3794) -> (-37.1512, -15.4099)
  line L94 (-37.1512, -15.4099) -> (-109.0802, -44.0021)
  line L95 (-109.0802, -44.0021) -> (-109.1866, -43.8009)
  line L96 (-109.1866, -43.8009) -> (-115.817, -20.4604)
  line L97 (-107.9955, -46.0543) -> (-107.6415, -46.5914)
  line L98 (-107.6415, -46.5914) -> (-35.1433, -19.1036)
  line L99 (-35.1433, -19.1036) -> (-33.1355, -22.7973)
  line L100 (-33.1355, -22.7973) -> (-97.7404, -65.3757)
  line L101 (-97.7404, -65.3757) -> (-95.6097, -67.4876)
  line L102 (-95.6097, -67.4876) -> (-30.4035, -25.9928)
  line L103 (-30.4035, -25.9928) -> (-27.6715, -29.1884)
  line L104 (-27.6715, -29.1884) -> (-82, -84)
  line L105 (-82, -84) -> (-79.7982, -86.0377)
  line L106 (-79.7982, -86.0377) -> (-24.3349, -31.7461)
  line L107 (-24.3349, -31.7461) -> (-20.9983, -34.3038)
  line L108 (-20.9983, -34.3038) -> (-62.5134, -99.4538)
  line L109 (-62.5134, -99.4538) -> (-59.7037, -100.5053)
  line L110 (-59.7037, -100.5053) -> (-17.2027, -36.1118)
  line L111 (-17.2027, -36.1118) -> (-13.4072, -37.9199)
  line L112 (-13.4072, -37.9199) -> (-40.5383, -110.4147)
  line L113 (-40.5383, -110.4147) -> (-40.0275, -110.5714)
  line L114 (-40.0275, -110.5714) -> (-40.5097, -110.4499)
  line L115 (-40.5097, -110.4499) -> (-62.5883, -99.6139)
  line L116 (-62.5883, -99.6139) -> (-81.9315, -84.4243)
  line L117 (-81.9315, -84.4243) -> (-97.6939, -65.5449)
  line L118 (-97.6939, -65.5449) -> (-107.9955, -46.0543)
  line L119 (-37.6242, -111.1769) -> (-9.3188, -38.8994)
  line L120 (-9.3188, -38.8994) -> (-5.2303, -39.8788)
  line L121 (-5.2303, -39.8788) -> (-16.8251, -116.2807)
  line L122 (-16.8251, -116.2807) -> (-13.8251, -116.2807)
  line L123 (-13.8251, -116.2807) -> (-1.0275, -39.9868)
  line L124 (-1.0275, -39.9868) -> (3.1753, -40.0948)
  line L125 (3.1753, -40.0948) -> (7.7901, -117.2299)
  line L126 (7.7901, -117.2299) -> (9.2805, -117.1408)
  line L127 (9.2805, -117.1408) -> (7.9166, -117.3778)
  line L128 (7.9166, -117.3778) -> (-16.6606, -116.4588)
  line L129 (-16.6606, -116.4588) -> (-37.6242, -111.1769)
  line L130 (10.7771, -116.8807) -> (7.3087, -39.3266)
  line L131 (7.3087, -39.3266) -> (11.4421, -38.5584)
  line L132 (11.4421, -38.5584) -> (32.1479, -113.1668)
  line L133 (32.1479, -113.1668) -> (32.1478, -113.1669)
  line L134 (32.1478, -113.1669) -> (10.7771, -116.8807)
  line L135 (34.941, -112.0464) -> (15.3254, -36.9477)
  line L136 (15.3254, -36.9477) -> (19.2088, -35.3369)
  line L137 (19.2088, -35.3369) -> (55.0494, -103.6389)
  line L138 (55.0494, -103.6389) -> (56.5162, -102.9753)
  line L139 (56.5162, -102.9753) -> (54.974, -104.01)
  line L140 (54.974, -104.01) -> (34.941, -112.0464)
  line L141 (57.6782, -102.1957) -> (22.6724, -32.9539)
  line L142 (22.6724, -32.9539) -> (26.136, -30.571)
  line L143 (26.136, -30.571) -> (75.334, -90.2327)
  line L144 (75.334, -90.2327) -> (76.0131, -89.6732)
  line L145 (76.0131, -89.6732) -> (75.3976, -90.3074)
  line L146 (75.3976, -90.3074) -> (57.6782, -102.1957)
  line L147 (77.5012, -88.1398) -> (29.0285, -27.52)
  line L148 (29.0285, -27.52) -> (31.9209, -24.4689)
  line L149 (31.9209, -24.4689) -> (91.7094, -73.4993)
  line L150 (91.7094, -73.4993) -> (77.5012, -88.1398)
  line L151 (114.1408, -28.313) -> (114.0793, -28.7426)
  line L152 (114.0793, -28.7426) -> (105.6105, -51.8329)
  line L153 (105.6105, -51.8329) -> (94.1326, -70.1008)
  line L154 (94.1326, -70.1008) -> (34.1158, -20.8832)
  line L155 (34.1158, -20.8832) -> (36.3108, -17.2975)
  line L156 (36.3108, -17.2975) -> (105.3224, -51.9766)
  line L157 (105.3224, -51.9766) -> (106.1029, -49.0799)
  line L158 (106.1029, -49.0799) -> (37.7122, -13.3338)
  line L159 (37.7122, -13.3338) -> (39.1136, -9.3701)
  line L160 (39.1136, -9.3701) -> (114.1408, -28.313)
  circle A1 centre (0, 0) radius 132.864
  circle A2 centre (0, 0) radius 126.4911
  constraint concentric A0 A1
  constraint concentric A0 A2
extrude "Extrude3" cut sketch "Sketch4" along normal blind 50 contours A1 in component "P1"
sketch "Sketch5" plane through (0, 0, 10) normal (0, 0, 1) x (-1, 0, 0) in component "P1"
  circle A0 centre (0, 0) radius 132.864
  line L0 (114.4294, -26.2951) -> (114.4825, -25.3611)
  line L1 (114.4825, -25.3611) -> (39.6603, -5.2016)
  line L2 (39.6603, -5.2016) -> (40.2071, -1.0331)
  line L3 (40.2071, -1.0331) -> (117.5488, -4.1953)
  line L4 (117.5488, -4.1953) -> (117.5623, -4.3961)
  line L5 (117.5623, -4.3961) -> (114.4294, -26.2951)
  line L6 (117.3513, -1.268) -> (117.3479, -1.2473)
  line L7 (117.3479, -1.2473) -> (39.8752, 3.1579)
  line L8 (39.8752, 3.1579) -> (39.5432, 7.349)
  line L9 (39.5432, 7.349) -> (115.9178, 19.9864)
  line L10 (115.9178, 19.9864) -> (117.3513, -1.268)
  line L11 (115.8188, 20.4539) -> (114.8879, 22.7863)
  line L12 (114.8879, 22.7863) -> (38.3472, 11.3794)
  line L13 (38.3472, 11.3794) -> (37.1512, 15.4099)
  line L14 (37.1512, 15.4099) -> (109.0294, 44.0983)
  line L15 (109.0294, 44.0983) -> (109.1866, 43.8009)
  line L16 (109.1866, 43.8009) -> (115.8188, 20.4539)
  line L17 (107.9951, 46.0551) -> (107.5799, 46.6822)
  line L18 (107.5799, 46.6822) -> (35.1433, 19.1036)
  line L19 (35.1433, 19.1036) -> (33.1355, 22.7973)
  line L20 (33.1355, 22.7973) -> (97.6947, 65.5432)
  line L21 (97.6947, 65.5432) -> (107.9951, 46.0551)
  line L22 (97.451, 65.8357) -> (95.589, 67.6691)
  line L23 (95.589, 67.6691) -> (30.4035, 25.9928)
  line L24 (30.4035, 25.9928) -> (27.6715, 29.1884)
  line L25 (27.6715, 29.1884) -> (81.9893, 84.355)
  line L26 (81.9893, 84.355) -> (97.451, 65.8357)
  line L27 (81.8802, 84.4645) -> (79.5062, 86.0276)
  line L28 (79.5062, 86.0276) -> (24.3349, 31.7461)
  line L29 (24.3349, 31.7461) -> (20.9983, 34.3038)
  line L30 (20.9983, 34.3038) -> (62.5297, 99.6426)
  line L31 (62.5297, 99.6426) -> (62.5883, 99.6139)
  line L32 (62.5883, 99.6139) -> (81.8802, 84.4645)
  line L33 (62.4555, 99.6791) -> (59.7198, 100.6884)
  line L34 (59.7198, 100.6884) -> (17.2027, 36.1118)
  line L35 (17.2027, 36.1118) -> (13.4072, 37.9199)
  line L36 (13.4072, 37.9199) -> (40, 110)
  line L37 (40, 110) -> (37.1974, 111.0702)
  line L38 (37.1974, 111.0702) -> (9.3188, 38.8994)
  line L39 (9.3188, 38.8994) -> (5.2303, 39.8788)
  line L40 (5.2303, 39.8788) -> (16.4634, 116.4661)
  line L41 (16.4634, 116.4661) -> (16.6606, 116.4588)
  line L42 (16.6606, 116.4588) -> (40.5097, 110.4499)
  line L43 (40.5097, 110.4499) -> (62.4555, 99.6791)
  line L44 (13.4779, 116.5778) -> (1.0275, 39.9868)
  line L45 (1.0275, 39.9868) -> (-3.1753, 40.0948)
  line L46 (-3.1753, 40.0948) -> (-7.3087, 117.1355)
  line L47 (-7.3087, 117.1355) -> (-10.2582, 116.5873)
  line L48 (-10.2582, 116.5873) -> (-7.3087, 39.3266)
  line L49 (-7.3087, 39.3266) -> (-11.4421, 38.5584)
  line L50 (-11.4421, 38.5584) -> (-32.2969, 113.1071)
  line L51 (-32.2969, 113.1071) -> (-32.1478, 113.1669)
  line L52 (-32.1478, 113.1669) -> (-7.9166, 117.3778)
  line L53 (-7.9166, 117.3778) -> (13.4779, 116.5778)
  line L54 (-35.0778, 111.9915) -> (-15.3254, 36.9477)
  line L55 (-15.3254, 36.9477) -> (-19.2088, 35.3369)
  line L56 (-19.2088, 35.3369) -> (-54.9971, 103.9945)
  line L57 (-54.9971, 103.9945) -> (-54.974, 104.01)
  line L58 (-54.974, 104.01) -> (-35.0778, 111.9915)
  line L59 (-57.4922, 102.3205) -> (-22.6724, 32.9539)
  line L60 (-22.6724, 32.9539) -> (-26.136, 30.571)
  line L61 (-26.136, 30.571) -> (-75.4486, 90.2548)
  line L62 (-75.4486, 90.2548) -> (-75.3976, 90.3074)
  line L63 (-75.3976, 90.3074) -> (-57.4922, 102.3205)
  line L64 (-77.5529, 88.0865) -> (-29.0285, 27.52)
  line L65 (-29.0285, 27.52) -> (-31.9209, 24.4689)
  line L66 (-31.9209, 24.4689) -> (-92.5771, 72.5765)
  line L67 (-92.5771, 72.5765) -> (-92.5259, 72.6579)
  line L68 (-92.5259, 72.6579) -> (-77.5529, 88.0865)
  line L69 (-93.8248, 70.5906) -> (-94.1009, 70.038)
  line L70 (-94.1009, 70.038) -> (-34.1158, 20.8832)
  line L71 (-34.1158, 20.8832) -> (-36.3108, 17.2975)
  line L72 (-36.3108, 17.2975) -> (-105.5702, 51.897)
  line L73 (-105.5702, 51.897) -> (-93.8248, 70.5906)
  line L74 (-114.0123, 28.9253) -> (-114.3288, 26.9982)
  line L75 (-114.3288, 26.9982) -> (-114.0793, 28.7426)
  line L76 (-114.0793, 28.7426) -> (-114.0123, 28.9253)
  line L77 (-113.9862, 28.9964) -> (-106.09, 50.5256)
  line L78 (-106.09, 50.5256) -> (-106.4726, 49.0659)
  line L79 (-106.4726, 49.0659) -> (-37.7122, 13.3338)
  line L80 (-37.7122, 13.3338) -> (-39.1136, 9.3701)
  line L81 (-39.1136, 9.3701) -> (-113.9862, 28.9964)
  line L82 (-114.4667, 26.0342) -> (-39.6603, 5.2016)
  line L83 (-39.6603, 5.2016) -> (-40.2071, 1.0331)
  line L84 (-40.2071, 1.0331) -> (-117.5048, 4.7978)
  line L85 (-117.5048, 4.7978) -> (-114.4667, 26.0342)
  line L86 (-117.4537, 2.7851) -> (-117.2992, 1.8519)
  line L87 (-117.2992, 1.8519) -> (-39.8752, -3.1579)
  line L88 (-39.8752, -3.1579) -> (-39.5432, -7.349)
  line L89 (-39.5432, -7.349) -> (-115.9178, -19.9864)
  line L90 (-115.9178, -19.9864) -> (-117.4537, 2.7851)
  line L91 (-115.817, -20.4604) -> (-114.8918, -22.7878)
  line L92 (-114.8918, -22.7878) -> (-38.3472, -11.3794)
  line L93 (-38.3472, -11.3794) -> (-37.1512, -15.4099)
  line L94 (-37.1512, -15.4099) -> (-109.0802, -44.0021)
  line L95 (-109.0802, -44.0021) -> (-109.1866, -43.8009)
  line L96 (-109.1866, -43.8009) -> (-115.817, -20.4604)
  line L97 (-107.9955, -46.0543) -> (-107.6415, -46.5914)
  line L98 (-107.6415, -46.5914) -> (-35.1433, -19.1036)
  line L99 (-35.1433, -19.1036) -> (-33.1355, -22.7973)
  line L100 (-33.1355, -22.7973) -> (-97.7404, -65.3757)
  line L101 (-97.7404, -65.3757) -> (-95.6097, -67.4876)
  line L102 (-95.6097, -67.4876) -> (-30.4035, -25.9928)
  line L103 (-30.4035, -25.9928) -> (-27.6715, -29.1884)
  line L104 (-27.6715, -29.1884) -> (-82, -84)
  line L105 (-82, -84) -> (-79.7982, -86.0377)
  line L106 (-79.7982, -86.0377) -> (-24.3349, -31.7461)
  line L107 (-24.3349, -31.7461) -> (-20.9983, -34.3038)
  line L108 (-20.9983, -34.3038) -> (-62.5134, -99.4538)
  line L109 (-62.5134, -99.4538) -> (-59.7037, -100.5053)
  line L110 (-59.7037, -100.5053) -> (-17.2027, -36.1118)
  line L111 (-17.2027, -36.1118) -> (-13.4072, -37.9199)
  line L112 (-13.4072, -37.9199) -> (-40.5383, -110.4147)
  line L113 (-40.5383, -110.4147) -> (-40.0275, -110.5714)
  line L114 (-40.0275, -110.5714) -> (-40.5097, -110.4499)
  line L115 (-40.5097, -110.4499) -> (-62.5883, -99.6139)
  line L116 (-62.5883, -99.6139) -> (-81.9315, -84.4243)
  line L117 (-81.9315, -84.4243) -> (-97.6939, -65.5449)
  line L118 (-97.6939, -65.5449) -> (-107.9955, -46.0543)
  line L119 (-37.6242, -111.1769) -> (-9.3188, -38.8994)
  line L120 (-9.3188, -38.8994) -> (-5.2303, -39.8788)
  line L121 (-5.2303, -39.8788) -> (-16.8251, -116.2807)
  line L122 (-16.8251, -116.2807) -> (-13.8251, -116.2807)
  line L123 (-13.8251, -116.2807) -> (-1.0275, -39.9868)
  line L124 (-1.0275, -39.9868) -> (3.1753, -40.0948)
  line L125 (3.1753, -40.0948) -> (7.7901, -117.2299)
  line L126 (7.7901, -117.2299) -> (9.2805, -117.1408)
  line L127 (9.2805, -117.1408) -> (7.9166, -117.3778)
  line L128 (7.9166, -117.3778) -> (-16.6606, -116.4588)
  line L129 (-16.6606, -116.4588) -> (-37.6242, -111.1769)
  line L130 (10.7771, -116.8807) -> (7.3087, -39.3266)
  line L131 (7.3087, -39.3266) -> (11.4421, -38.5584)
  line L132 (11.4421, -38.5584) -> (32.1479, -113.1668)
  line L133 (32.1479, -113.1668) -> (32.1478, -113.1669)
  line L134 (32.1478, -113.1669) -> (10.7771, -116.8807)
  line L135 (34.941, -112.0464) -> (15.3254, -36.9477)
  line L136 (15.3254, -36.9477) -> (19.2088, -35.3369)
  line L137 (19.2088, -35.3369) -> (55.0494, -103.6389)
  line L138 (55.0494, -103.6389) -> (56.5162, -102.9753)
  line L139 (56.5162, -102.9753) -> (54.974, -104.01)
  line L140 (54.974, -104.01) -> (34.941, -112.0464)
  line L141 (57.6782, -102.1957) -> (22.6724, -32.9539)
  line L142 (22.6724, -32.9539) -> (26.136, -30.571)
  line L143 (26.136, -30.571) -> (75.334, -90.2327)
  line L144 (75.334, -90.2327) -> (76.0131, -89.6732)
  line L145 (76.0131, -89.6732) -> (75.3976, -90.3074)
  line L146 (75.3976, -90.3074) -> (57.6782, -102.1957)
  line L147 (77.5012, -88.1398) -> (29.0285, -27.52)
  line L148 (29.0285, -27.52) -> (31.9209, -24.4689)
  line L149 (31.9209, -24.4689) -> (91.7094, -73.4993)
  line L150 (91.7094, -73.4993) -> (77.5012, -88.1398)
  line L151 (114.1408, -28.313) -> (114.0793, -28.7426)
  line L152 (114.0793, -28.7426) -> (105.6105, -51.8329)
  line L153 (105.6105, -51.8329) -> (94.1326, -70.1008)
  line L154 (94.1326, -70.1008) -> (34.1158, -20.8832)
  line L155 (34.1158, -20.8832) -> (36.3108, -17.2975)
  line L156 (36.3108, -17.2975) -> (105.3224, -51.9766)
  line L157 (105.3224, -51.9766) -> (106.1029, -49.0799)
  line L158 (106.1029, -49.0799) -> (37.7122, -13.3338)
  line L159 (37.7122, -13.3338) -> (39.1136, -9.3701)
  line L160 (39.1136, -9.3701) -> (114.1408, -28.313)
  circle A1 centre (0, 0) radius 132.864
  circle A2 centre (0, 0) radius 124.6547
  constraint concentric A0 A1
  constraint concentric A0 A2
extrude "Extrude4" add sketch "Sketch5" along normal blind 35 contours A0 A1 in component "P1"
component "P1" placed x (1, 0, 0) y (0, 1, 0) z (0, 0, 1) at (0, 0, 0)
